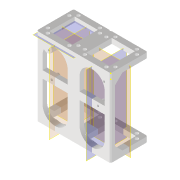
# Autodesk Inventor part: 40_Cube_XY_Table_Aliexpress_naked_electronicsmount_base
Saved by Autodesk Inventor 2022 (Build 260153000, 153)
## iProperties
Created: 2022-02-11
Part Number: 40_Cube_XY_Table_Aliexpress_naked_electronicsmount_base
Material: Generic
Document SubType Name: Modeling
Designer: wanghaoran
Density: 1 g/cm^3
Appearance: Default
Catalog Web Link: isPrinted
Vendor: openUC2
Mass: 36.1859 g
Surface Area: 194.638 cm^2
Volume: 36.1859 cm^3
Author: wanghaoran
Autodesk Inventor part; units mm, degrees
ref_plane "YZ Plane" through (0, 0, 0) normal (1, 0, 0) x (0, 1, 0)
ref_plane "XZ Plane" through (0, 0, 0) normal (0, 1, 0) x (-1, 0, 0)
sketch "Sketch1" plane through (0, 0, 0) normal (0, 1, 0) x (-1, 0, 0)
  line L0 (0, 0) -> (49.8, 0)
  line L1 (49.8, 0) -> (49.8, -49.8)
  line L2 (49.8, -49.8) -> (0, -49.8)
  line L3 (0, -49.8) -> (0, 0)
  line L4 (7.8, -7.8) -> (42, -7.8)
  line L5 (42, -7.8) -> (42, -42)
  line L6 (42, -42) -> (7.8, -42)
  line L7 (7.8, -42) -> (7.8, -7.8)
  line L8 (42, -7.8) -> (7.8, -7.8)
  line L9 (42, -42) -> (49.8, -42)
  line L10 (49.8, -42) -> (49.8, -7.8)
  line L11 (49.8, -7.8) -> (42, -7.8)
  line L12 (42, -7.8) -> (42, -42)
  dimension "d0" = 49.8
  dimension "d1" = 49.8
  dimension "d2" = 7.8
  constraints: 26 end point, 6 parallel, 3 horizontal, 3 perpendicular, 1 point on line, 3 other
  measures "d0" distance of L1.end L2.end
  measures "d1" distance of L0.end L1.end
  measures "d2" distance between parallel lines of L3 L7
extrude "Extrusion1" add sketch "Sketch1" along normal blind 7 contours L0 L1 L11 L4 L7 L6 L9 L2 L3
sketch "Sketch3" plane through (0, 0, 0) normal (0, -1, 0) x (1, 0, 0)
  line L0 (-49.8, 0) -> (0, 0) projected
  line L1 (-49.8, -49.8) -> (-49.8, 0) projected
  line L2 (0, 0) -> (-49.8, 0)
  line L3 (-49.8, 0) -> (-49.8, -4.55)
  line L4 (-49.8, -4.55) -> (0, -4.55)
  line L5 (0, -4.55) -> (0, 0)
  line L6 (-7.8, -42) -> (-7.8, -7.8) projected
  line L7 (0, -49.8) -> (-7.8, -49.8)
  line L8 (-7.8, -49.8) -> (-7.8, -42)
  line L9 (-7.8, -42) -> (0, -42)
  line L10 (0, -42) -> (0, -49.8)
  line L11 (0, -49.8) -> (-49.8, -49.8) projected
  line L12 (-42, -7.8) -> (-42, -42) projected
  line L13 (-49.8, -49.8) -> (-42, -49.8)
  line L14 (-42, -49.8) -> (-42, -42)
  line L15 (-42, -42) -> (-49.8, -42)
  line L16 (-49.8, -42) -> (-49.8, -49.8)
  line L17 (-7.8, -4.55) -> (-42, -4.55) projected
  line L18 (-49.8, -4.55) -> (-42, -4.55)
  line L19 (-42, -4.55) -> (-42, -6)
  line L20 (-42, -6) -> (-49.8, -6)
  line L21 (-49.8, -6) -> (-49.8, -4.55)
  line L22 (0, -4.55) -> (-7.8, -4.55)
  line L23 (-7.8, -4.55) -> (-7.8, -6)
  line L24 (-7.8, -6) -> (0, -6)
  line L25 (0, -6) -> (0, -4.55)
  line L26 (-42, -6) -> (-7.8, -6)
  line L27 (-7.8, -6) -> (-7.8, -4.55)
  line L28 (-7.8, -4.55) -> (-42, -4.55)
  line L29 (-42, -4.55) -> (-42, -6)
  point P0 (-49.8, -6)
  point P1 (-49.8, 0)
  dimension "d57" = 0
  dimension "d58" = 6
  dimension "d59" = 6
  constraints: 48 end point, 12 parallel, 6 horizontal, 6 perpendicular, 3 point on line
  measures "d57" distance between parallel lines of L17 L4
  measures "d58" distance between parallel lines of L20 L0
  measures "d59" distance between parallel lines of L24 L0
extrude "Extrusion2" add sketch "Sketch3" against normal blind 98 contours L0 L5 L4 L1 | L4 L19 L20 L1 | L25 L24 L23 L4 | L4 L23 L26 L19
sketch "Sketch4" plane through (-49.8, 0, 0) normal (0, 0, 1) x (1, 0, 0)
  line L0 (8, 80.5) -> (41.8, 80.5)
  line L1 (41.8, 80.5) -> (41.8, 23)
  line L2 (41.8, 23) -> (8, 23)
  line L3 (8, 23) -> (8, 80.5)
  circle A0 centre (24.9, 80.5) radius 16.9
  circle A1 centre (24.9, 23) radius 16.9
  line L4 (49.8, 0) -> (49.8, 98) projected
  line L5 (0, 0) -> (0, 98) projected
  line L6 (0, 0) -> (49.8, 0) projected
  line L7 (0, 98) -> (49.8, 98) projected
  point P0 (8, 80.5)
  point P1 (8, 80.5)
  point P2 (8, 23)
  point P3 (16.4, 34)
  point P4 (33.4, 34)
  point P5 (8, 23)
  dimension "d125" = 49.8
  dimension "d126" = 24.9
  dimension "d127" = 33.8
  dimension "d128" = 23
  dimension "d129" = 17.5
  constraints: 8 end point, 2 midpoint, 2 parallel, 1 horizontal, 1 perpendicular, 6 other
  measures "d125" distance between parallel lines of L4 L5
  measures "d126" distance from line of point (24.9, 80.5) L5
  measures "d127" distance between parallel lines of L1 L3
  measures "d128" distance from line of L6 point (24.9, 23)
  measures "d129" distance from line of L7 point (24.9, 80.5)
extrude "Extrusion3" cut sketch "Sketch4" against normal up to surface (42 mm away) contours A0 L0 | A0 L1 A1 L3 | L0 A0 | A1 L2 | L2 A1
fillet "Fillet1" radius 2 2 edges at (0, 49, 0) (0, 3.5, -49.8)
ref_plane "Arbeitsebene1" through (-24.9, 7, -4.55) normal (-1, 0, 0) x (0, 0, 1)
ref_plane "Arbeitsebene2" through (-47.8, 0, -24.9) normal (0, 0, 1) x (1, 0, 0)
sketch "Skizze8" plane through (0, 0, 0) normal (0, -1, 0) x (1, 0, 0)
  line L0 (-49.9, -29.9) -> (-49.9, -47.9) projected
  arc A0 (-49.9, -47.9) -> (-47.9, -49.9) centre (-47.9, -47.9) ccw projected
  line L1 (-30.0511, -49.9) -> (-47.9, -49.9) projected
  line L2 (-30.0511, -49.9) -> (-30.0509, -49.1742) projected
  arc A1 (-30.0509, -49.1742) -> (-30.2806, -48.8498) centre (-30.3999, -49.1778) ccw projected
  arc A2 (-31.9947, -46.7407) -> (-30.2806, -48.8498) centre (-29.84, -46.7407) ccw projected
  line L3 (-31.9947, -46.7407) -> (-31.9947, -46.6009) projected
  arc A3 (-29.8434, -44.4498) -> (-31.9947, -46.6009) centre (-29.8435, -46.6009) ccw projected
  line L4 (-29.8434, -44.4498) -> (-19.9598, -44.4503) projected
  arc A4 (-17.81, -46.6004) -> (-19.9598, -44.4503) centre (-19.96, -46.6003) ccw projected
  line L5 (-17.81, -46.6004) -> (-17.81, -46.7408) projected
  arc A5 (-19.52, -48.8451) -> (-17.81, -46.7408) centre (-19.9599, -46.7406) ccw projected
  arc A6 (-19.52, -48.8451) -> (-19.7498, -49.1739) centre (-19.3996, -49.1739) ccw projected
  line L6 (-19.7498, -49.1739) -> (-19.7495, -49.9) projected
  line L7 (-1.9, -49.9) -> (-19.7495, -49.9) projected
  arc A7 (-1.9, -49.9) -> (0.1, -47.9) centre (-1.9, -47.9) ccw projected
  line L8 (0.1, -47.9) -> (0.1, -30.0511) projected
  line L9 (0.1, -30.0511) -> (-0.6258, -30.0509) projected
  arc A8 (-0.6258, -30.0509) -> (-0.9502, -30.2806) centre (-0.6222, -30.3999) ccw projected
  arc A9 (-3.0593, -31.9947) -> (-0.9502, -30.2806) centre (-3.0593, -29.84) ccw projected
  line L10 (-3.0593, -31.9947) -> (-3.1991, -31.9947) projected
  arc A10 (-5.3502, -29.8434) -> (-3.1991, -31.9947) centre (-3.1991, -29.8435) ccw projected
  line L11 (-5.3502, -29.8434) -> (-5.3497, -19.9598) projected
  arc A11 (-3.1996, -17.81) -> (-5.3497, -19.9598) centre (-3.1997, -19.96) ccw projected
  line L12 (-3.1996, -17.81) -> (-3.0592, -17.81) projected
  arc A12 (-0.9549, -19.52) -> (-3.0592, -17.81) centre (-3.0594, -19.9599) ccw projected
  arc A13 (-0.9549, -19.52) -> (-0.6261, -19.7498) centre (-0.6261, -19.3996) ccw projected
  line L13 (-0.6261, -19.7498) -> (0.1, -19.7495) projected
  line L14 (0.1, -19.7495) -> (0.1, -1.9) projected
  arc A14 (0.1, -1.9) -> (-1.9, 0.1) centre (-1.9, -1.9) ccw projected
  line L15 (-19.9, 0.1) -> (-1.9, 0.1) projected
  line L16 (-19.9, 0.1) -> (-19.9, 0.9263) projected
  arc A15 (-19.56, 1.4) -> (-19.9, 0.9263) centre (-19.4, 0.9263) ccw projected
  arc A16 (-19.56, 1.4) -> (-17.96, 3.3596) centre (-19.96, 3.3596) ccw projected
  line L17 (-17.96, 3.3596) -> (-17.96, 3.5) projected
  arc A17 (-17.96, 3.5) -> (-19.96, 5.5) centre (-19.96, 3.5) ccw projected
  line L18 (-19.96, 5.5) -> (-29.84, 5.5) projected
  arc A18 (-29.84, 5.5) -> (-31.84, 3.5) centre (-29.84, 3.5) ccw projected
  line L19 (-31.84, 3.5) -> (-31.84, 3.3596) projected
  arc A19 (-31.84, 3.3596) -> (-30.24, 1.4) centre (-29.84, 3.3596) ccw projected
  arc A20 (-29.9, 0.9263) -> (-30.24, 1.4) centre (-30.4, 0.9263) ccw projected
  line L20 (-29.9, 0.9263) -> (-29.9, 0.1) projected
  line L21 (-47.9, 0.1) -> (-29.9, 0.1) projected
  arc A21 (-47.9, 0.1) -> (-49.9, -1.9) centre (-47.9, -1.9) ccw projected
  line L22 (-49.9, -1.9) -> (-49.9, -19.9) projected
  line L23 (-49.9, -19.9) -> (-50.7263, -19.9) projected
  arc A22 (-51.2, -19.56) -> (-50.7263, -19.9) centre (-50.7263, -19.4) ccw projected
  arc A23 (-51.2, -19.56) -> (-53.1596, -17.96) centre (-53.1596, -19.96) ccw projected
  line L24 (-53.1596, -17.96) -> (-53.3, -17.96) projected
  arc A24 (-53.3, -17.96) -> (-55.3, -19.96) centre (-53.3, -19.96) ccw projected
  line L25 (-55.3, -19.96) -> (-55.3, -29.84) projected
  arc A25 (-55.3, -29.84) -> (-53.3, -31.84) centre (-53.3, -29.84) ccw projected
  line L26 (-53.3, -31.84) -> (-53.1596, -31.84) projected
  arc A26 (-53.1596, -31.84) -> (-51.2, -30.24) centre (-53.1596, -29.84) ccw projected
  arc A27 (-50.7263, -29.9) -> (-51.2, -30.24) centre (-50.7263, -30.4) ccw projected
  line L27 (-50.7263, -29.9) -> (-49.9, -29.9) projected
  arc A28 (-49.9, -26.2329) -> (-49.9, -23.7671) centre (-46.2, -25) ccw projected
  line L28 (-49.9, -26.2329) -> (-49.9, -23.7671) projected
  circle A29 centre (-25, -3.6) radius 3.9 projected
  line L29 (-7.6, -40.2) -> (-7.6, -9.6) projected
  arc A30 (-9.6, -42.2) -> (-7.6, -40.2) centre (-9.6, -40.2) ccw projected
  line L30 (-9.6, -42.2) -> (-40.2, -42.2) projected
  arc A31 (-42.2, -40.2) -> (-40.2, -42.2) centre (-40.2, -40.2) ccw projected
  line L31 (-42.2, -9.6) -> (-42.2, -40.2) projected
  arc A32 (-40.2, -7.6) -> (-42.2, -9.6) centre (-40.2, -9.6) ccw projected
  line L32 (-40.2, -7.6) -> (-9.6, -7.6) projected
  arc A33 (-7.6, -9.6) -> (-9.6, -7.6) centre (-9.6, -9.6) ccw projected
  circle A34 centre (-44.8, -5) radius 2.4 projected
  circle A35 centre (-39.35, -4.35) radius 2.45 projected
  circle A36 centre (-45.45, -10.45) radius 2.45 projected
  circle A37 centre (-4.35, -10.45) radius 2.45 projected
  circle A38 centre (-10.45, -4.35) radius 2.45 projected
  circle A39 centre (-5, -5) radius 2.4 projected
  circle A40 centre (-45.45, -39.35) radius 2.45 projected
  circle A41 centre (-39.35, -45.45) radius 2.45 projected
  circle A42 centre (-44.8, -44.8) radius 2.4 projected
  circle A43 centre (-4.35, -39.35) radius 2.45 projected
  circle A44 centre (-10.45, -45.45) radius 2.45 projected
  circle A45 centre (-5, -44.8) radius 2.4 projected
  point P0 (0, 0)
hole "Bohrung1" at (-45.45, 0, -39.35) at (-45.45, 0, -10.45) at (-4.35, 0, -10.45) at (-4.35, 0, -39.35) at (-10.45, 0, -45.45) at (-39.35, 0, -45.45) at (-39.35, 0, -4.35) at (-10.45, 0, -4.35) direction (0, 1, 0) diameter 4.8 depth 12 tip angle 118
sketch "Skizze10" plane through (0, 98, 0) normal (0, 1, 0) x (1, 0, 0)
  arc A0 (-25.6984, 4.55) -> (-24.1016, 4.55) centre (-24.9, 3.4) ccw projected
  point P0 (0, 0)
sketch "Skizze14" plane through (0, 98, 0) normal (0, 1, 0) x (1, 0, 0)
  circle A0 centre (-10.45, 45.45) radius 2.3 projected
  circle A1 centre (-4.35, 10.45) radius 2.3 projected
  circle A2 centre (-45.45, 39.35) radius 2.3 projected
  circle A3 centre (-45.45, 10.45) radius 2.3 projected
  circle A4 centre (-4.35, 39.35) radius 2.3 projected
  circle A5 centre (-39.35, 45.45) radius 2.3 projected
  line L0 (-9.3, 42) -> (-40.5, 42) projected
  line L1 (-9.3, 7.8) -> (-9.3, 42) projected
  line L2 (-9.7, 7.8) -> (-9.3, 7.8) projected
  line L3 (-9.7, 4.35) -> (-9.7, 7.8) projected
  line L4 (-12.75, 4.35) -> (-9.7, 4.35) projected
  arc A6 (-12.7413, 4.55) -> (-12.75, 4.35) centre (-10.45, 4.35) ccw projected
  line L5 (-37.0587, 4.55) -> (-12.7413, 4.55) projected
  arc A7 (-37.05, 4.35) -> (-37.0587, 4.55) centre (-39.35, 4.35) ccw projected
  line L6 (-40.1, 4.35) -> (-37.05, 4.35) projected
  line L7 (-40.1, 7.8) -> (-40.1, 4.35) projected
  line L8 (-40.5, 7.8) -> (-40.1, 7.8) projected
  line L9 (-40.5, 42) -> (-40.5, 7.8) projected
  line L10 (-49.8, 49.8) -> (-2, 49.8) projected
  arc A8 (-49.8, 49.8) -> (-49.8, 47.8) centre (-47.8, 47.8) ccw projected
  line L11 (-49.8, 2) -> (-49.8, 47.8) projected
  arc A9 (-49.8, 2) -> (-47.8, 0) centre (-47.8, 2) ccw projected
  line L12 (-2, 0) -> (-47.8, 0) projected
  arc A10 (-2, 0) -> (0, 2) centre (-2, 2) ccw projected
  line L13 (0, 47.8) -> (0, 2) projected
  arc A11 (0, 47.8) -> (-2, 49.8) centre (-2, 47.8) ccw projected
  line L14 (-2, 49.8) -> (-49.8, 49.8) projected
  line L15 (-7.8, 42) -> (-7.8, 7.8) projected
  arc A12 (-49.8, 49.8) -> (-49.8, 47.8) centre (-47.8, 47.8) ccw projected
  arc A13 (0, 47.8) -> (-2, 49.8) centre (-2, 47.8) ccw projected
  arc A14 (-40.5, 47.75) -> (-42.4975, 49.8) centre (-42.4975, 47.8018) ccw
  line L16 (-40.5, 47.75) -> (-42.4975, 49.8) construction
  line L17 (-40.5, 47.75) -> (-37.6377, 47.75) construction
  arc A15 (-7.25, 49.8) -> (-9.3, 47.75) centre (-7.25, 47.75) ccw
  line L18 (-9.3, 47.75) -> (-7.25, 49.8) construction
  line L19 (-9.3, 47.75) -> (-6.4009, 47.75) construction
  line L20 (-42, 7.8) -> (-42, 42) projected
  line L21 (-40.5, 42) -> (-40.5, 49.8)
  line L22 (-9.3, 42) -> (-9.3, 49.8)
  circle A16 centre (-10.45, 4.35) radius 2.4 projected
  circle A17 centre (-39.35, 4.35) radius 2.4 projected
  arc A18 (-37.6072, 6) -> (-41.0928, 6) centre (-39.35, 4.35) ccw projected
  line L23 (-30.3415, 6) -> (-30.3415, 7.8) projected
  line L24 (-30.3415, 7.8) -> (-49.8, 7.8) projected
  line L25 (-49.8, 42) -> (-7.8, 42) projected
  line L26 (-7.8, 42) -> (-7.8, 7.8) projected
  line L27 (-7.8, 7.8) -> (-19.4585, 7.8) projected
  line L28 (-19.4585, 7.8) -> (-19.4585, 6) projected
  arc A19 (-8.7072, 6) -> (-12.1928, 6) centre (-10.45, 4.35) ccw projected
  line L29 (0, 6) -> (0, 47.8) projected
  arc A20 (0, 47.8) -> (-2, 49.8) centre (-2, 47.8) ccw projected
  line L30 (-2, 49.8) -> (-49.8, 49.8) projected
  line L31 (-49.8, 7.8) -> (-49.8, 6) projected
  circle A21 centre (-10.45, 45.45) radius 2.4 projected
  circle A22 centre (-4.35, 10.45) radius 2.4 projected
  circle A23 centre (-4.35, 39.35) radius 2.4 projected
  circle A24 centre (-39.35, 45.45) radius 2.4 projected
  line L32 (-30.3415, 6) -> (-30.3415, 7.8) projected
  line L33 (-30.3415, 7.8) -> (-19.4585, 7.8)
  line L34 (-8.7072, 6) -> (0, 6) projected
  line L35 (-49.8, 6) -> (-41.0928, 6) projected
  line L36 (-37.6072, 6) -> (-30.3415, 6) projected
  line L37 (-19.4585, 6) -> (-12.1928, 6) projected
  line L38 (-49.8, 6) -> (-49.8, 0) projected
  line L39 (-49.8, 0) -> (-2, 0) projected
  line L40 (-49.8, 49.8) -> (-49.8, 42) projected
  point P0 (0, 0)
  point P1 (-7.8, 6)
  point P2 (-42, 6)
  point P3 (-7.25, 49.8)
  point P4 (-7.8, 4.55)
  point P5 (-42, 4.55)
  point P6 (-40.5, 47.8536)
  point P7 (-37.73, 4.55)
  point P8 (-9.4763, 7.8)
  point P9 (-40.3235, 7.8)
  point P10 (-37.73, 6.1208)
  point P11 (-7.25, 49.8)
  point P12 (-49.8, 47.8)
  point P13 (-7.8, 7.8)
  point P14 (-9.4763, 7.8)
  point P15 (-40.3235, 7.8)
  dimension "d121" = 134.257
  dimension "d122" = 45
  constraints: 14 end point, 6 point on line, 4 point on circle, 3 horizontal, 2 centre point, 2 equal length, 2 perpendicular, 2 tangent, 3 other
  measures "d121" angle of L17 L16
  measures "d122" angle of L19 L18
ref_plane "Arbeitsebene3" through (-49.8, 100, -49.8) normal (0, -1, 0) x (1, 0, 0)
extrude "Extrusion7" add sketch "Skizze14" along normal blind 7 contours A0 L22 | A0 L22 A21 | L22 A0 | A0 L22 A21 | L21 A24 L25 L11 L40 L10 A14 | A21 L22 L0 L21 A24 L10 | L22 A15 L10 A11 L13 L34 A16 L3 L2 L27 L15 L25 A21 | L22 L10 A15 | L21 A14 L10 | L8 L7 A17 L35 L11 L24 | A24 L21 A5 | L21 A5 A24 | L3 A16 L37 L28 L27 | L24 L23 L36 A17 L7 | L21 A5 | A5 L21 | L28 L37 A16 L5 A17 L36 L23 L33 | L13 A10 L12 A9 L11 L35 A17 L5 A16 L34 | A9 L39 L38 | A1 | A4 | A22 | A23
sketch "Skizze24" plane through (0, 0, -2) normal (1, 0, 0) x (0, 0, -1)
  line L0 (45.8, 7) -> (45.8, 0) projected
  line L1 (4, 7) -> (45.8, 7) projected
  line L2 (4, 7) -> (4, 98) projected
  line L3 (0, 0) -> (0, 105) projected
  line L4 (0, 0) -> (45.8, 0) projected
  line L5 (14, 7) -> (4, 17)
  line L6 (4, 23) -> (4, 12.0816) projected
  line L7 (14, 7) -> (28.1421, 7) construction
  line L8 (4, 7) -> (4, 98) projected
  line L9 (4, 88) -> (14, 98)
  line L10 (40, 98) -> (5.8, 98) projected
  line L11 (4, 88) -> (18.1421, 88) construction
  line L12 (4, 98) -> (45.8, 98) projected
  line L13 (45.8, 98) -> (45.8, 105) projected
  line L14 (0, 105) -> (45.8, 105) projected
  point P0 (-2, 0)
  point P1 (5.8, 98)
  dimension "d150" = 135
  dimension "d151" = 45
  dimension "d152" = 10
  dimension "d153" = 10
  constraints: 8 end point, 4 point on line, 2 equal length, 2 horizontal
  measures "d150" angle of L7 L5
  measures "d151" angle of L11 L9
  measures "d152" distance from line of L2 L5.start
  measures "d153" distance from line of L9.end L8
extrude "Extrusion16" add sketch "Skizze24" against normal up to surface (8 mm away) contours L1 L2 L5 | L2 L12 L10 L9
mirror "Spiegeln4" about plane through (-49.8, 0, -7.8) normal (-1, 0, 0) of "Extrusion1", "Extrusion2", "Extrusion3", "Fillet1", "Bohrung1", "Extrusion7", "Extrusion16"
sketch "Skizze25" plane through (-2, 0, 0) normal (0, 0, 1) x (1, 0, 0)
  circle A0 centre (-14.985, 58.53) radius 1.5 projected
  circle A1 centre (-16.335, 24.24) radius 1.6 projected
  circle A2 centre (-81.105, 90.28) radius 1.6 projected
  circle A3 centre (-77.295, 57.895) radius 1.6 projected
  arc A4 (-55.8, 80.5) -> (-89.6, 80.5) centre (-72.7, 80.5) ccw projected
  line L0 (-89.6, 23) -> (-89.6, 80.5) projected
  circle A5 centre (-6.81, 90.915) radius 1.6 projected
  arc A6 (-87.7105, 88.2649) -> (-78.895, 96.2236) centre (-82.9709, 91.8766) ccw
  line L1 (-89.6, 80.5) -> (-89.6, 23) projected
  line L2 (-55.8, 23) -> (-55.8, 80.5) projected
  line L3 (-89.6, 62.895) -> (-55.8, 62.895)
  line L4 (-55.8, 62.895) -> (-55.8, 52.895)
  line L5 (-55.8, 52.895) -> (-89.6, 52.895)
  line L6 (-89.6, 52.895) -> (-89.6, 62.895)
  line L7 (-39.8, 80.5) -> (-39.8, 23) projected
  line L8 (-6, 23) -> (-6, 80.5) projected
  line L9 (-39.8, 62.895) -> (-6, 62.895)
  line L10 (-6, 62.895) -> (-6, 52.895)
  line L11 (-6, 52.895) -> (-39.8, 52.895)
  line L12 (-39.8, 52.895) -> (-39.8, 62.895)
  point P0 (2, 0)
  point P1 (-55.8, 62.895)
  point P2 (-6, 62.895)
  dimension "d156" = 5
  dimension "d157" = 5
  constraints: 16 end point, 6 point on line, 4 parallel, 4 point on circle, 2 horizontal, 2 perpendicular, 1 centre point
  measures "d156" distance from line of A3.centre L3
  measures "d157" distance from line of A3.centre L5
extrude "Extrusion17" add sketch "Skizze25" against normal up to surface (6 mm away) contours A0 | A2 | A6 A4 | L2 L5 L0 L3 | L9 L8 L11 L7
sketch "Skizze26" plane through (-12.1928, 98, -6) normal (0, 0, -1) x (-1, 0, 0)
  circle A0 centre (70.9122, -7.72) radius 1.6 projected
  circle A1 centre (6.1422, -73.76) radius 1.6 projected
  circle A2 centre (-3.3828, -7.085) radius 1.6 projected
  circle A3 centre (67.1022, -40.105) radius 1.6 projected
  circle A4 centre (4.7922, -39.47) radius 1.5 projected
  circle A5 centre (-3.3828, -7.085) radius 3.6
  circle A6 centre (70.9122, -7.72) radius 3.6
  circle A7 centre (67.1022, -40.105) radius 3.6
  circle A8 centre (4.7922, -39.47) radius 3.5
  circle A9 centre (6.1422, -73.76) radius 3.6
  point P0 (-12.1928, -98)
  dimension "d160" = 2
  dimension "d161" = 2
  dimension "d162" = 2
  dimension "d163" = 2
  dimension "d164" = 2
  constraints: 5 centre point
  measures "d160" radial gap between concentric circles of A2 A5
  measures "d161" radial gap between concentric circles of A0 A6
  measures "d162" radial gap between concentric circles of A3 A7
  measures "d163" radial gap between concentric circles of A4 A8
  measures "d164" radial gap between concentric circles of A1 A9
extrude "Extrusion18" add sketch "Skizze26" along normal blind 3 contours A0 | A2 | A3 | A4 | A5 | A6 | A7 | A8
sketch "Skizze27" plane through (-2, 0, 0) normal (0, 0, 1) x (1, 0, 0)
  circle A0 centre (-81.105, 90.28) radius 1.6 projected
  circle A1 centre (-6.81, 90.915) radius 1.6 projected
  circle A2 centre (-14.985, 58.53) radius 1.5 projected
  circle A3 centre (-77.295, 57.895) radius 1.6 projected
  point P0 (2, 0)
hole "Bohrung6" at (-8.81, 90.915, 0) at (-16.985, 58.53, 0) at (-79.295, 57.895, 0) at (-83.105, 90.28, 0) direction (0, 0, -1) diameter 2.8 end through all
sketch "Skizze28" plane through (-12.1928, 98, -9) normal (0, 0, -1) x (-1, 0, 0)
  line L0 (75.9922, -89) -> (-7.1928, -89) projected
  line L1 (75.9922, -2.5835) -> (75.9922, -89) projected
  line L2 (-7.1928, -2.64) -> (75.9922, -2.5835) projected
  line L3 (-7.1928, -89) -> (-7.1928, -2.64) projected
  circle A0 centre (-2.1128, -82.65) radius 0.5 projected
  circle A1 centre (-2.1128, -80.11) radius 0.5 projected
  circle A2 centre (-2.1128, -77.57) radius 0.5 projected
  circle A3 centre (-2.1128, -72.49) radius 0.5 projected
  circle A4 centre (-2.1128, -69.95) radius 0.5 projected
  circle A5 centre (-2.1128, -67.41) radius 0.5 projected
  circle A6 centre (6.1422, -73.76) radius 1.6 projected
  circle A7 centre (-2.1828, -62.33) radius 0.5 projected
  circle A8 centre (-2.1828, -59.79) radius 0.5 projected
  circle A9 centre (-2.1828, -57.25) radius 0.5 projected
  circle A10 centre (-2.1828, -52.155) radius 0.5 projected
  circle A11 centre (-2.1828, -49.615) radius 0.5 projected
  circle A12 centre (-2.1828, -47.075) radius 0.5 projected
  circle A13 centre (4.8722, -59.155) radius 0.5 projected
  circle A14 centre (7.4122, -59.155) radius 0.5 projected
  circle A15 centre (4.8722, -54.075) radius 0.5 projected
  circle A16 centre (7.4122, -54.075) radius 0.5 projected
  circle A17 centre (13.7622, -58.52) radius 0.55 projected
  circle A18 centre (4.8722, -48.36) radius 0.5 projected
  circle A19 centre (7.4122, -48.36) radius 0.5 projected
  circle A20 centre (13.7622, -51.86) radius 0.55 projected
  circle A21 centre (13.7622, -44.875) radius 0.55 projected
  circle A22 centre (15.0322, -82.015) radius 0.5 projected
  circle A23 centre (17.5722, -82.015) radius 0.5 projected
  circle A24 centre (20.1122, -82.015) radius 0.5 projected
  circle A25 centre (25.1922, -82.015) radius 0.5 projected
  circle A26 centre (27.7322, -82.015) radius 0.5 projected
  circle A27 centre (30.2722, -82.015) radius 0.5 projected
  circle A28 centre (27.0972, -71.855) radius 0.5 projected
  circle A29 centre (29.6372, -71.855) radius 0.5 projected
  circle A30 centre (32.1772, -71.855) radius 0.5 projected
  circle A31 centre (16.3022, -58.52) radius 0.55 projected
  circle A32 centre (18.8422, -58.52) radius 0.55 projected
  circle A33 centre (16.3022, -51.86) radius 0.55 projected
  circle A34 centre (18.8422, -51.86) radius 0.55 projected
  circle A35 centre (16.3022, -44.875) radius 0.55 projected
  circle A36 centre (18.8422, -44.875) radius 0.55 projected
  circle A37 centre (27.1072, -46.43) radius 0.5 projected
  circle A38 centre (29.6472, -46.43) radius 0.5 projected
  circle A39 centre (32.1872, -46.43) radius 0.5 projected
  circle A40 centre (-4.2078, -39.47) radius 0.8 projected
  circle A41 centre (-2.2078, -43.97) radius 1.25 projected
  circle A42 centre (-1.2078, -39.47) radius 1.15 projected
  circle A43 centre (-2.2078, -34.97) radius 1.25 projected
  circle A44 centre (1.3262, -31.85) radius 0.4 projected
  circle A45 centre (1.3262, -29.31) radius 0.4 projected
  circle A46 centre (1.3262, -26.77) radius 0.4 projected
  circle A47 centre (4.7922, -39.47) radius 1.5 projected
  circle A48 centre (14.0262, -31.85) radius 0.4 projected
  circle A49 centre (14.0262, -29.31) radius 0.4 projected
  circle A50 centre (14.0262, -26.77) radius 0.4 projected
  circle A51 centre (1.3262, -24.23) radius 0.4 projected
  circle A52 centre (1.3262, -21.69) radius 0.4 projected
  circle A53 centre (1.3262, -19.15) radius 0.4 projected
  circle A54 centre (1.3262, -16.61) radius 0.4 projected
  circle A55 centre (-3.3828, -7.085) radius 1.6 projected
  circle A56 centre (1.3262, -14.07) radius 0.4 projected
  circle A57 centre (4.2372, -7.466) radius 0.5 projected
  circle A58 centre (14.0262, -24.23) radius 0.4 projected
  circle A59 centre (14.0262, -21.69) radius 0.4 projected
  circle A60 centre (14.0262, -19.15) radius 0.4 projected
  circle A61 centre (14.0262, -16.61) radius 0.4 projected
  circle A62 centre (6.7772, -7.466) radius 0.5 projected
  circle A63 centre (9.3172, -7.466) radius 0.5 projected
  circle A64 centre (14.0262, -14.07) radius 0.4 projected
  circle A65 centre (11.8572, -7.466) radius 0.5 projected
  circle A66 centre (18.4612, -31.85) radius 0.4 projected
  circle A67 centre (18.4612, -29.31) radius 0.4 projected
  circle A68 centre (18.4612, -26.77) radius 0.4 projected
  circle A69 centre (31.1612, -31.85) radius 0.4 projected
  circle A70 centre (31.1612, -29.31) radius 0.4 projected
  circle A71 centre (31.1612, -26.77) radius 0.4 projected
  circle A72 centre (18.4612, -24.23) radius 0.4 projected
  circle A73 centre (18.4612, -21.69) radius 0.4 projected
  circle A74 centre (18.4612, -19.15) radius 0.4 projected
  circle A75 centre (18.4612, -16.61) radius 0.4 projected
  circle A76 centre (18.4612, -14.07) radius 0.4 projected
  circle A77 centre (21.1282, -7.339) radius 0.5 projected
  circle A78 centre (23.6682, -7.339) radius 0.5 projected
  circle A79 centre (31.1612, -24.23) radius 0.4 projected
  circle A80 centre (31.1612, -21.69) radius 0.4 projected
  circle A81 centre (31.1612, -19.15) radius 0.4 projected
  circle A82 centre (31.1612, -16.61) radius 0.4 projected
  circle A83 centre (26.2082, -7.339) radius 0.5 projected
  circle A84 centre (28.7482, -7.339) radius 0.5 projected
  circle A85 centre (31.1612, -14.07) radius 0.4 projected
  circle A86 centre (35.9872, -82.015) radius 0.5 projected
  circle A87 centre (38.5272, -82.015) radius 0.5 projected
  circle A88 centre (41.0672, -82.015) radius 0.5 projected
  circle A89 centre (34.7172, -71.855) radius 0.5 projected
  circle A90 centre (37.2572, -71.855) radius 0.5 projected
  circle A91 centre (39.7972, -71.855) radius 0.5 projected
  circle A92 centre (42.3372, -71.855) radius 0.5 projected
  circle A93 centre (45.5122, -82.015) radius 0.5 projected
  circle A94 centre (48.0522, -82.015) radius 0.5 projected
  circle A95 centre (50.5922, -82.015) radius 0.5 projected
  circle A96 centre (44.8772, -71.855) radius 0.5 projected
  circle A97 centre (47.4172, -71.855) radius 0.5 projected
  circle A98 centre (49.9572, -71.855) radius 0.5 projected
  circle A99 centre (52.4972, -71.855) radius 0.5 projected
  circle A100 centre (34.7272, -46.43) radius 0.5 projected
  circle A101 centre (37.2672, -46.43) radius 0.5 projected
  circle A102 centre (39.8072, -46.43) radius 0.5 projected
  circle A103 centre (42.3472, -46.43) radius 0.5 projected
  circle A104 centre (44.8872, -46.43) radius 0.5 projected
  circle A105 centre (47.4272, -46.43) radius 0.5 projected
  circle A106 centre (49.9672, -46.43) radius 0.5 projected
  circle A107 centre (52.5072, -46.43) radius 0.5 projected
  circle A108 centre (55.6722, -82.015) radius 0.5 projected
  circle A109 centre (58.2122, -82.015) radius 0.5 projected
  circle A110 centre (60.7522, -82.015) radius 0.5 projected
  circle A111 centre (55.0372, -71.855) radius 0.5 projected
  circle A112 centre (57.5772, -71.855) radius 0.5 projected
  circle A113 centre (60.1172, -71.855) radius 0.5 projected
  circle A114 centre (62.6572, -71.855) radius 0.5 projected
  circle A115 centre (65.8322, -82.015) radius 0.5 projected
  circle A116 centre (68.3722, -82.015) radius 0.5 projected
  circle A117 centre (70.9122, -82.015) radius 0.5 projected
  circle A118 centre (65.1972, -71.855) radius 0.5 projected
  circle A119 centre (67.7372, -71.855) radius 0.5 projected
  circle A120 centre (70.2772, -71.855) radius 0.5 projected
  circle A121 centre (72.8172, -71.855) radius 0.5 projected
  circle A122 centre (55.0472, -46.43) radius 0.5 projected
  circle A123 centre (57.5872, -46.43) radius 0.5 projected
  circle A124 centre (60.1272, -46.43) radius 0.5 projected
  circle A125 centre (62.6672, -46.43) radius 0.5 projected
  circle A126 centre (65.2072, -46.43) radius 0.5 projected
  circle A127 centre (67.7472, -46.43) radius 0.5 projected
  circle A128 centre (70.2872, -46.43) radius 0.5 projected
  circle A129 centre (72.8272, -46.43) radius 0.5 projected
  circle A130 centre (35.9872, -31.85) radius 0.4 projected
  circle A131 centre (35.9872, -29.31) radius 0.4 projected
  circle A132 centre (35.9872, -26.77) radius 0.4 projected
  circle A133 centre (48.6872, -31.85) radius 0.4 projected
  circle A134 centre (48.6872, -29.31) radius 0.4 projected
  circle A135 centre (48.6872, -26.77) radius 0.4 projected
  circle A136 centre (35.9872, -24.23) radius 0.4 projected
  circle A137 centre (35.9872, -21.69) radius 0.4 projected
  circle A138 centre (35.9872, -19.15) radius 0.4 projected
  circle A139 centre (35.9872, -16.61) radius 0.4 projected
  circle A140 centre (35.9872, -14.07) radius 0.4 projected
  circle A141 centre (39.2892, -7.339) radius 0.5 projected
  circle A142 centre (41.8292, -7.339) radius 0.5 projected
  circle A143 centre (48.6872, -24.23) radius 0.4 projected
  circle A144 centre (48.6872, -21.69) radius 0.4 projected
  circle A145 centre (48.6872, -19.15) radius 0.4 projected
  circle A146 centre (48.6872, -16.61) radius 0.4 projected
  circle A147 centre (48.6872, -14.07) radius 0.4 projected
  circle A148 centre (44.3692, -7.339) radius 0.5 projected
  circle A149 centre (46.9092, -7.339) radius 0.5 projected
  circle A150 centre (53.7672, -31.85) radius 0.4 projected
  circle A151 centre (53.7672, -29.31) radius 0.4 projected
  circle A152 centre (53.7672, -26.77) radius 0.4 projected
  circle A153 centre (67.1022, -40.105) radius 1.6 projected
  circle A154 centre (66.4672, -31.85) radius 0.4 projected
  circle A155 centre (66.4672, -29.31) radius 0.4 projected
  circle A156 centre (66.4672, -26.77) radius 0.4 projected
  circle A157 centre (53.7672, -24.23) radius 0.4 projected
  circle A158 centre (53.7672, -21.69) radius 0.4 projected
  circle A159 centre (53.7672, -19.15) radius 0.4 projected
  circle A160 centre (53.7672, -16.61) radius 0.4 projected
  circle A161 centre (53.7672, -14.07) radius 0.4 projected
  circle A162 centre (56.5612, -7.339) radius 0.5 projected
  circle A163 centre (59.1012, -7.339) radius 0.5 projected
  circle A164 centre (61.6412, -7.339) radius 0.5 projected
  circle A165 centre (66.4672, -24.23) radius 0.4 projected
  circle A166 centre (66.4672, -21.69) radius 0.4 projected
  circle A167 centre (66.4672, -19.15) radius 0.4 projected
  circle A168 centre (66.4672, -16.61) radius 0.4 projected
  circle A169 centre (66.4672, -14.07) radius 0.4 projected
  circle A170 centre (64.1812, -7.339) radius 0.5 projected
  circle A171 centre (70.9122, -7.72) radius 1.6 projected
  line L4 (77.9922, -91) -> (-9.1928, -91)
  line L5 (-9.1928, -91) -> (-9.1928, -0.6414)
  line L6 (-9.1928, -0.6414) -> (77.9922, -0.5821)
  line L7 (77.9922, -0.5821) -> (77.9922, -91)
  point P0 (-12.1928, -98)
  dimension "d174" = 2
  constraints: 8 end point, 3 other
  measures "d174" distance between parallel lines of L1 L7
extrude "Extrusion19" cut sketch "Skizze28" along normal through all contours L0 L3 L2 L1 | A0 | A1 | A2 | A3 | A4 | A5 | A6 | A7 | A8 | A9 | A10 | A11 | A12 | A13 | A14 | A15 | A16 | A17 | A18 | A19 | A20 | A21 | A22 | A23 | A24 | A25 | A26 | A27 | A28 | A29 | A30 | A31 | A32 | A33 | A34 | A35 | A36 | A37 | A38 | A39 | A40 | A41 | A42 | A43 | A44 | A45 | A46 | A47 | A48 | A49 | A50 | A51 | A52 | A53 | A54 | A55 | A56 | A57 | A58 | A59 | A60 | A61 | A62 | A63 | A64 | A65 | A66 | A67 | A68 | A69 | A70 | A71 | A72 | A73 | A74 | A75 | A76 | A77 | A78 | A79 | A80 | A81 | A82 | A83 | A84 | A85 | A86 | A87 | A88 | A89 | A90 | A91 | A92 | A93 | A94 | A95 | A96 | A97 | A98 | A99 | A100 | A101 | A102 | A103 | A104 | A105 | A106 | A107 | A108 | A109 | A110 | A111 | A112 | A113 | A114 | A115 | A116 | A117 | A118 | A119 | A120 | A121 | A122 | A123 | A124 | A125 | A126 | A127 | A128 | A129 | A130 | A131 | A132 | A133 | A134 | A135 | A136 | A137 | A138 | A139 | A140 | A141 | A142 | A143 | A144 | A145 | A146 | A147 | A148 | A149 | A150 | A151 | A152 | A153 | A154 | A155 | A156 | A157 | A158 | A159 | A160 | A161 | A162 | A163 | A164 | A165 | A166 | A167 | A168 | A169 | A170 | A171 | L4 L5 L6 L7
sketch "Skizze29" plane through (0, 105, 0) normal (0, 1, 0) x (1, 0, 0)
  point P0 (0, 0)
ref_plane "Arbeitsebene4" through (-49.8, 100, -49.8) normal (0, 1, 0) x (-1, 0, 0)
ref_plane "Arbeitsebene5" through (-74.7, 7, -4.55) normal (-1, 0, 0) x (0, 0, 1)
ref_plane "Arbeitsebene6" through (-51.8, 0, -24.9) normal (0, 0, -1) x (-1, 0, 0)
equation "\"d59\" = d58"
body "Solid1"
